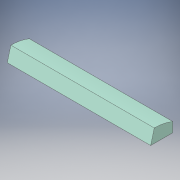
# Autodesk Inventor part: spacebar-keycap_mockup_cherrymx
Saved by Autodesk Inventor 2016 (Build 200138000, 138)
## iProperties
Created: 2016-12-10
Part Number: spacebar-keycap_mockup_cherrymx
Material: Generic
Document SubType Name: Modeling
Designer: Cemra JC
Density: 1 g/cm^3
Appearance: Default
Author: Cemra JC
Autodesk Inventor part; units mm, degrees
ref_plane "YZ Plane" through (0, 0, 0) normal (1, 0, 0) x (0, 1, 0)
ref_plane "XZ Plane" through (0, 0, 0) normal (0, 1, 0) x (-1, 0, 0)
ref_plane "XY Plane" through (0, 0, 0) normal (0, 0, 1) x (1, 0, 0)
sketch "Spacebar base" plane through (0, 0, 0) normal (0, 1, 0) x (-1, 0, 0)
  line L0 (56.875, 8.75) -> (-56.875, 8.75)
  line L1 (-56.875, 8.75) -> (-56.875, -8.75)
  line L2 (-56.875, -8.75) -> (56.875, -8.75)
  line L3 (56.875, -8.75) -> (56.875, 8.75)
  line L4 (56.875, 8.75) -> (-56.875, -8.75) construction
  line L5 (-56.875, 8.75) -> (56.875, -8.75) construction
  point P0 (0, 0)
  dimension "d0" = 113.75
  dimension "d1" = 17.5
  constraints: 12 end point, 2 midpoint, 2 parallel, 1 horizontal, 1 perpendicular
  measures "d0" distance of L2.end L1.end
  measures "d1" distance of L1.end L0.end
extrude "Spacebar Bulk" add sketch "Spacebar base" along normal blind 11
sketch "Curve Profile" plane through (56.875, 0, 8.75) normal (1, 0, 0) x (0, 0, -1)
  line L0 (0, 0) -> (17.5, 0) projected
  line L1 (0, 0) -> (2.9474, 11)
  line L2 (0, 11) -> (17.5, 11) projected
  line L3 (17.5, 0) -> (17.5, 11) projected
  arc A0 (17.5, 8) -> (2.9474, 11) centre (2.9474, -25.7962) ccw
  line L4 (0, 0) -> (0, 11) projected
  line L5 (17.5, 8) -> (17.5, 0)
  line L6 (17.5, 0) -> (0, 0)
  point P0 (8.75, 0)
  dimension "d4" = 15
  dimension "d9" = 8
  constraints: 6 end point, 2 collinear, 2 point on circle, 2 point on line, 1 centre point, 1 tangent
  measures "d4" angle of L1 L4
  measures "d9" distance of L0.end L5.start
extrude "Curve Cutaway" cut sketch "Curve Profile" against normal up to surface (113.75 mm away) contours L1 A0 L3 L0 keep common part
shell "Inner Shell" thickness 1.5 removed faces 1 at (18.9583, 0, -2.9167)
ref_plane "PoleBase Plane" through (55.375, 9.4814, 4.6566) normal (0, 0.9994728, -0.0324682) x (-1, 0, 0)
sketch "Center Circle" plane through (55.375, 9.4814, 4.6566) normal (0, 0.9994728, -0.0324682) x (-1, 0, 0)
  circle A0 centre (55.375, -4.9619) radius 2.65
  dimension "d11" = 5.3
  constraints: 1 centre point, 1 coincident
  measures "d11" diameter of A0
extrude "Pole Extrusion" add sketch "Center Circle" against normal up to surface surface through (0, 0, 0) normal (0, 1, 0)
sketch "Sketch4" plane through (0, 0, 0) normal (0, -1, 0) x (1, 0, 0)
  line L0 (-2.075, 0.6) -> (2.075, 0.6)
  line L1 (2.075, 0.6) -> (2.075, -0.6)
  line L2 (2.075, -0.6) -> (-2.075, -0.6)
  line L3 (-2.075, -0.6) -> (-2.075, 0.6)
  line L4 (-2.075, 0.6) -> (2.075, -0.6) construction
  line L5 (2.075, 0.6) -> (-2.075, -0.6) construction
  line L6 (0.6, 2.075) -> (-0.6, 2.075)
  line L7 (-0.6, 2.075) -> (-0.6, -2.075)
  line L8 (-0.6, -2.075) -> (0.6, -2.075)
  line L9 (0.6, -2.075) -> (0.6, 2.075)
  line L10 (0.6, 2.075) -> (-0.6, -2.075) construction
  line L11 (-0.6, 2.075) -> (0.6, -2.075) construction
  point P0 (0, 0)
  dimension "d14" = 4.15
  dimension "d15" = 1.2
  dimension "d16" = 1.2
  dimension "d17" = 4.15
  constraints: 24 end point, 4 midpoint, 4 parallel, 2 horizontal, 2 perpendicular
  measures "d14" distance of L1.end L2.end
  measures "d15" distance of L0.end L1.end
  measures "d16" distance of L8.end L7.end
  measures "d17" distance of L7.end L6.end
extrude "Extrusion4" cut sketch "Sketch4" against normal blind 5
equation "\"d0\" = b_space"
equation "\"d1\" = k_width"
equation "\"d10\" = k_wthick"
equation "\"d11\" = k_poledia"
equation "\"d14\" = k_cmxl"
equation "\"d15\" = k_cmxw"
equation "\"d16\" = k_cmxw"
equation "\"d17\" = k_cmxl"
equation "\"k_width\" = 17.5"
equation "\"k_height\" = 16.5"
equation "\"k_height_t\" = 16"
equation "\"k_taper1\" = 1.5"
equation "\"k_taper2\" = 0.5"
equation "\"k_staper\" = 1"
equation "\"k_sradius\" = 4"
equation "\"k_ltaper\" = 1.5"
equation "\"k_lradius\" = 6"
equation "\"k_radius\" = 6"
equation "\"k_wthick\" = 1.5"
equation "\"k_ribthick\" = 1.5"
equation "\"k_ribheight\" = 5"
equation "\"k_poleoff\" = 2.1875"
equation "\"k_poledia\" = 5.3"
equation "\"k_cmxw\" = 1.2"
equation "\"k_cmxl\" = 4.15"
equation "\"s_bwidth\" = 14.4"
equation "\"s_poleh\" = 3.6"
equation "\"s_polebw\" = 5.4"
equation "\"s_polebl\" = 7.45"
equation "\"b_pad\" = 1"
equation "\"b_tab\" = 26.25"
equation "\"b_caps\" = 30.625"
equation "\"b_lshift\" = 39.375"
equation "\"b_rshift\" = 48.125"
equation "\"b_ctrl\" = 21.875"
equation "\"b_space\" = 113.75"
equation "\"b_width\" = 277.5"
equation "\"b_height\" = 75"
equation "\"k_taper_wide\" = 1.5"
equation "\"k_height_low\" = 15"
equation "\"k_taper_thin\" = 0.0001"
equation "\"k_shortening\" = 4.5"
equation "\"k_cmxd\" = 4"
body "Solid1"
